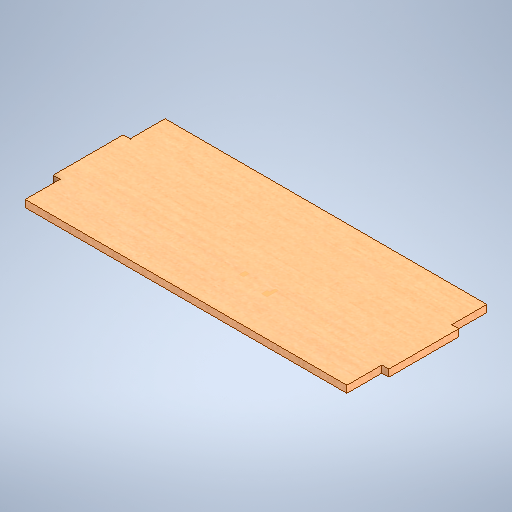
# Autodesk Inventor part: Tapa2
Saved by Autodesk Inventor 2025 (Build 290162000, 162)
## iProperties
Created: 2024-11-02
Part Number: Tapa2
Material: Wood (Cherry)
Document SubType Name: Sheet Metal
Designer: g.marin
Density: 0.63 g/cm^3
Sheet Metal Rule: Default
Appearance: Cherry - Natural Low Gloss
Author: g.marin
Autodesk Inventor part; units mm, degrees
ref_plane "YZ Plane" through (0, 0, 0) normal (1, 0, 0) x (0, 1, 0)
ref_plane "XZ Plane" through (0, 0, 0) normal (0, 1, 0) x (-1, 0, 0)
ref_plane "XY Plane" through (0, 0, 0) normal (0, 0, 1) x (1, 0, 0)
sketch "Sketch1" plane through (0, 0, 0) normal (0, 1, 0) x (-1, 0, 0)
  line L0 (-115, 50) -> (115, 50)
  line L1 (115, 50) -> (115, -50)
  line L2 (115, -50) -> (-115, -50)
  line L3 (-115, -50) -> (-115, 50)
  line L4 (-115, 50) -> (115, -50) construction
  line L5 (115, 50) -> (-115, -50) construction
  line L6 (0, 50) -> (0, -50) construction
  line L7 (115, 25) -> (120, 25)
  line L8 (120, 25) -> (120, -25)
  line L9 (120, -25) -> (115, -25)
  line L10 (115, -25) -> (115, 25)
  line L11 (-115, 25) -> (-120, 25)
  line L12 (-120, 25) -> (-120, -25)
  line L13 (-120, -25) -> (-115, -25)
  point P0 (0, 0)
  point P1 (-115, -25)
  dimension "d0" = 100
  dimension "d1" = 230
  dimension "d2" = 50
  dimension "d3" = 5
  dimension "d4" = 25
  constraints: 28 end point, 4 midpoint, 4 parallel, 4 symmetric about line, 2 horizontal, 2 perpendicular, 1 point on line
  measures "d0" distance of L0.end L1.end
  measures "d1" distance of L1.end L2.end
  measures "d2" distance of L7.end L8.end
  measures "d3" distance of L8.end L9.end
  measures "d4" vertical distance of L7.end L0.end
extrude "Extrusion1" add sketch "Sketch1" along normal blind 5
equation "\"BendRadius\" = Thickness"
equation "\"BendReliefWidth\" = Thickness"
equation "\"BendReliefDepth\" = 0.5 * Thickness"
equation "\"CornerReliefSize\" = 4 * Thickness"
equation "\"MinimumRemnant\" = 2 * Thickness"
equation "\"TransitionRadius\" = BendRadius"
equation "\"JacobiRadiusSize\" = BendRadius"
equation "\"GapSize\" = Thickness"
equation "\"Thickness\" = 3.048"
body "Solid1"
